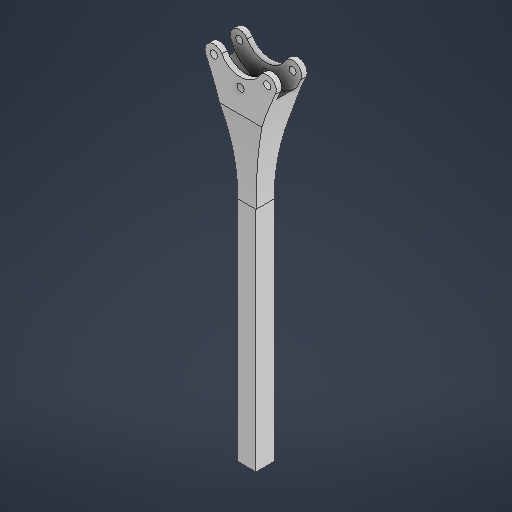
# Autodesk Inventor part: lower_leg
Saved by Autodesk Inventor 2026 (Build 300175000, 175)
## iProperties
Created: 2025-07-14
Part Number: lower_leg
Material: Generic
Document SubType Name: Modeling
Designer: User
Density: 1 g/cm^3
Appearance: Default
Author: User
Autodesk Inventor part; units mm, degrees
ref_plane "YZ Plane" through (0, 0, 0) normal (1, 0, 0) x (0, 1, 0)
ref_plane "XZ Plane" through (0, 0, 0) normal (0, 1, 0) x (-1, 0, 0)
sketch "Sketch1" plane through (0, 0, 0) normal (0, 0, 1) x (1, 0, 0)
  circle A0 centre (0, 0) radius 12 construction
  circle A1 centre (0, 0) radius 22 construction
  line L0 (0, 0) -> (-22, 0) construction
  line L1 (0, -12) -> (0, -22) construction
  circle A2 centre (0, 0) radius 17 construction
  arc A3 (-15.9748, -5.8143) -> (15.9748, -5.8143) centre (0, 0) ccw construction
  line L2 (-19.0526, -11) -> (0, 0) construction
  line L3 (0, 0) -> (19.0526, -11) construction
  line L4 (0, 0) -> (23.7434, 0) construction
  arc A4 (-14.7224, -8.5) -> (14.7224, -8.5) centre (0, 0) ccw construction
  arc A5 (-10.3923, -6) -> (10.3923, -6) centre (0, 0) ccw
  arc A6 (-10.3923, -6) -> (-19.0526, -11) centre (-14.7224, -8.5) ccw
  arc A7 (19.0526, -11) -> (10.3923, -6) centre (14.7224, -8.5) ccw
  circle A8 centre (0, -17) radius 2
  circle A9 centre (-14.7224, -8.5) radius 2
  circle A10 centre (14.7224, -8.5) radius 2
  line L5 (0, 0) -> (0, -250) construction
  line L6 (5, -195) -> (5, -21.4243)
  line L7 (-5, -195) -> (-5, -21.4243)
  line L8 (5, -195) -> (5, -200)
  line L9 (5, -200) -> (-5, -200)
  line L10 (-5, -200) -> (-5, -195)
  arc A11 (-19.0526, -11) -> (-5, -21.4243) centre (0, 0) ccw
  arc A12 (5, -21.4243) -> (19.0526, -11) centre (0, 0) ccw
  dimension "d0" = 24
  dimension "d1" = 10
  dimension "d4" = 30
  dimension "d5" = 30
  dimension "d6" = 4
  dimension "d7" = 4
  dimension "d8" = 4
  dimension "d9" = 250
  constraints: 22 end point, 21 point on circle, 12 centre point, 4 coincident, 3 vertical, 2 horizontal, 2 point on line, 2 tangent, 1 parallel, 1 vertical alignment, 2 other
  measures "d4" angle of L0 L2
  measures "d5" angle of L4 L3
  measures "d6" diameter of A8
  measures "d7" diameter of A9
  measures "d8" diameter of A10
  measures "d9" distance of L5.end L5.start
extrude "Extrusion1" add sketch "Sketch1" along normal blind 17
fillet "Fillet1" radius 150 2 edges at (5, -21.4243, 8.5) (-5, -21.4243, 8.5)
sketch "Sketch2" plane through (-5, -200, 0) normal (-1, 0, 0) x (0, 0, 1)
  line L0 (0, 0) -> (17, 0) projected
  line L1 (8.5, 0) -> (13.5, 0)
  line L2 (8.5, 0) -> (3.5, 0)
  line L3 (3.5, 0) -> (3.5, 170)
  line L4 (0, 196.5) -> (17, 196.5) projected
  line L5 (3.5, 170) -> (-8.9088, 170)
  line L6 (-8.9088, 170) -> (-8.9088, 0)
  line L7 (-8.9088, 0) -> (0, 0)
  line L8 (8.5, 0) -> (8.5, -9.0953) construction
  line L9 (17, 0) -> (0, 0)
  line L10 (13.5, 0) -> (13.5, 170)
  line L11 (13.5, 170) -> (25.9088, 170)
  line L12 (25.9088, 170) -> (25.9088, 0)
  line L13 (25.9088, 0) -> (17, 0)
  point P0 (0, 200)
  dimension "d14" = 5
  dimension "d15" = 5
  dimension "d16" = 170
  constraints: 24 end point, 5 symmetric about line, 3 point on line, 2 perpendicular, 1 collinear, 1 horizontal, 1 midpoint, 1 vertical
  measures "d14" distance of L1.start L1.end
  measures "d15" distance of L1.start L2.end
  measures "d16" distance of L2.end L3.end
extrude "Extrusion2" cut sketch "Sketch2" along normal mid plane 47.7625
fillet "Fillet2" radius 283.8 2 edges at (0, -30, 13.5) (0, -30, 3.5)
ref_plane "Work Plane1" through (0, 0, 14) normal (0, 0, 1) x (1, 0, 0)
sketch "Sketch5" plane through (0, 0, 14) normal (0, 0, 1) x (1, 0, 0)
  circle A0 centre (0, 0) radius 23
  dimension "d23" = 46
  constraints: 1 centre point, 1 coincident
  measures "d23" diameter of A0
extrude "Extrusion3" cut sketch "Sketch5" against normal blind 11
body "Solid1"
